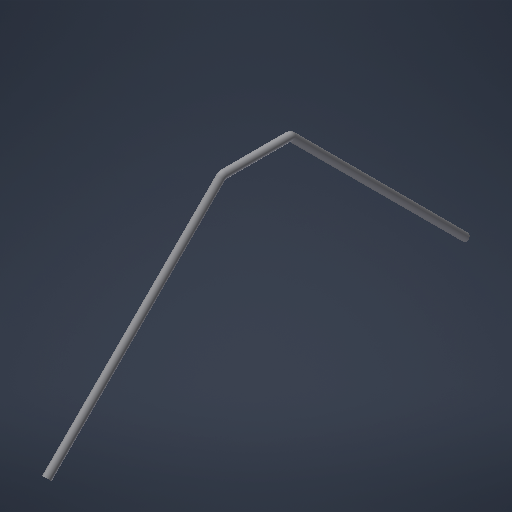
# Autodesk Inventor part: Pieza2
Saved by Autodesk Inventor 2026 (Build 300175000, 175)
## iProperties
Created: 2025-06-27
Part Number: Pieza2
Material: Generic
Document SubType Name: Modeling
Designer: usuario
Density: 1 g/cm^3
Appearance: Default
Author: usuario
Autodesk Inventor part; units mm, degrees
ref_plane "YZ Plane" through (0, 0, 0) normal (1, 0, 0) x (0, 1, 0)
ref_plane "XZ Plane" through (0, 0, 0) normal (0, 1, 0) x (-1, 0, 0)
ref_plane "XY Plane" through (0, 0, 0) normal (0, 0, 1) x (1, 0, 0)
sketch "Boceto1" plane through (0, 0, 0) normal (1, 0, 0) x (0, 1, 0)
  line L0 (-91.0046, 108.7546) -> (-0.5858, 18.3358)
  line L1 (0, 16.9216) -> (0, -16.9216)
  line L2 (-0.5858, -18.3358) -> (-91.0046, -108.7546)
  arc A0 (0, 16.9216) -> (-0.5858, 18.3358) centre (-2, 16.9216) ccw
  arc A1 (-0.5858, -18.3358) -> (0, -16.9216) centre (-2, -16.9216) ccw
  point P0 (0, 0)
  point P1 (0, 17.75)
  point P2 (0, -17.75)
  point P3 (0, 0)
  dimension "d0" = 128.7
  dimension "d1" = 128.7
  dimension "d2" = 35.5
  dimension "d3" = 2
  constraints: 6 end point, 4 point on circle, 4 point on line, 4 tangent, 2 centre point, 2 coincident, 1 equal radius, 1 midpoint, 1 perpendicular, 1 vertical, 1 vertical alignment
  measures "d0" distance of L0.start point (0, 17.75)
  measures "d1" distance of point (0, -17.75) L2.end
  measures "d2" distance of point (0, 17.75) point (0, -17.75)
  measures "d3" radius of A0
sketch "Boceto2" plane through (0, 0, 0) normal (0, 0, 1) x (1, 0, 0)
  circle A0 centre (0, 0) radius 2
  dimension "d4" = 4
  constraints: 1 centre point, 1 coincident
  measures "d4" diameter of A0
sweep "Barrido1" add profiles "Boceto2" path "Boceto1"
